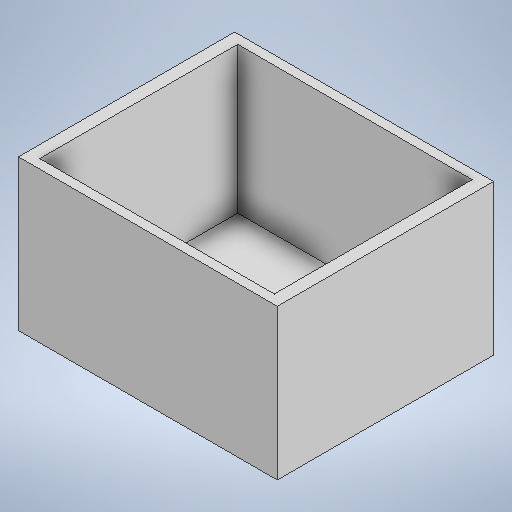
# Autodesk Inventor part: Olkasse
Saved by Autodesk Inventor 2025.2 (Build 292293000, 293)
## iProperties
Created: 2025-03-19
Part Number: Olkasse
Material: Generic
Document SubType Name: Modeling
Designer: Mathias B. Kampp
Density: 1 g/cm^3
Appearance: Default
Author: Mathias B. Kampp
Autodesk Inventor part; units mm, degrees
ref_plane "YZ Plane" through (0, 0, 0) normal (1, 0, 0) x (0, 1, 0)
ref_plane "XZ Plane" through (0, 0, 0) normal (0, 1, 0) x (-1, 0, 0)
ref_plane "XY Plane" through (0, 0, 0) normal (0, 0, 1) x (1, 0, 0)
sketch "Sketch1" plane through (0, 0, 0) normal (0, 1, 0) x (-1, 0, 0)
  line L0 (0, 0) -> (-425, 0)
  line L1 (-425, 0) -> (-425, -355)
  line L2 (-425, -355) -> (0, -355)
  line L3 (0, -355) -> (0, 0)
  line L4 (-20, -15) -> (-405, -15)
  line L5 (-405, -15) -> (-405, -340)
  line L6 (-405, -340) -> (-20, -340)
  line L7 (-20, -340) -> (-20, -15)
  dimension "d0" = 425
  dimension "d1" = 355
  dimension "d2" = 385
  dimension "d3" = 325
  constraints: 16 end point, 4 parallel, 2 horizontal, 2 perpendicular
  measures "d0" distance of L2.end L1.end
  measures "d1" distance of L1.end L0.end
  measures "d2" distance of L6.end L5.end
  measures "d3" distance of L5.end L4.end
extrude "Extrusion1" add sketch "Sketch1" along normal blind 247
sketch "Sketch2" plane through (0, 0, 0) normal (0, -1, 0) x (1, 0, 0)
  line L0 (0, -355) -> (0, 0) projected
  line L1 (425, 0) -> (425, -355) projected
  line L2 (0, 0) -> (425, 0)
  line L3 (425, 0) -> (425, -355)
  line L4 (425, -355) -> (0, -355)
  line L5 (0, -355) -> (0, 0)
  constraints: 8 end point, 2 parallel, 1 horizontal, 1 perpendicular
extrude "Extrusion2" add sketch "Sketch2" against normal blind 7
body "Solid1"
